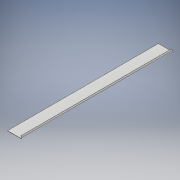
# Autodesk Inventor part: sideplate part 2
Saved by Autodesk Inventor 2018 (Build 220112000, 112)
## iProperties
Created: 2018-06-05
Part Number: sideplate part 2
Material: Generic
Document SubType Name: Sheet Metal
Designer: John Viljoen
Density: 1 g/cm^3
Sheet Metal Rule: Default_mm
Appearance: Default
Author: John Viljoen
Autodesk Inventor part; units mm, degrees
ref_plane "YZ Plane" through (0, 0, 0) normal (1, 0, 0) x (0, 1, 0)
ref_plane "XZ Plane" through (0, 0, 0) normal (0, 1, 0) x (-1, 0, 0)
ref_plane "XY Plane" through (0, 0, 0) normal (0, 0, 1) x (1, 0, 0)
sketch "Sketch1" plane through (0, 0, 0) normal (0, 0, 1) x (1, 0, 0)
  line L0 (0, 0) -> (29.621, 0)
  line L1 (29.621, 0) -> (29.621, 338.525)
  line L2 (29.621, 338.525) -> (0, 338.525)
  line L3 (0, 338.525) -> (0, 0)
  dimension "d0" = 29.621
  dimension "d1" = 338.525
  measures "d0" distance of L2.end L1.end
  measures "d1" distance of L1.end L0.end
extrude "Plate1" add sketch "Sketch1" along normal blind 0.5
sketch "Sketch2" plane through (31.0058, 338.525, 2.5764) normal (0.9232102, 0, 0.3842953) x (0, 1, 0)
  line L0 (-338.525, 0) -> (0, 0)
  line L1 (0, 0) -> (0, 3.0011)
  line L2 (0, 3.0011) -> (-338.525, 3.0011)
  line L3 (-338.525, 3.0011) -> (-338.525, 0)
  constraints: 6 end point, 1 horizontal, 1 perpendicular, 1 vertical
edge flange "Flange1" height 6 angle 112.6 thickness 0.5 bend radius 1.5 thickness toward (0.9232102, 0, 0.3842953) relief straight relief width 0.5 relief depth 0.25 edges at (29.621, 169.2625, 0.5) wall of the first edge with corners at (31.0058, 0, 2.5764) (31.0058, 338.525, 2.5764) (29.8525, 338.525, 5.3471) (29.8525, 0, 5.3471)
bend "Bend1"
corner "Corner1"
equation "\"d2\" = Thickness"
equation "\"d3\" = BendReliefWidth"
equation "\"d4\" = BendReliefDepth"
equation "\"d5\" = MinimumRemnant"
equation "\"d6\" = TransitionRadius"
equation "\"d10\" = CornerReliefSize"
equation "\"d11\" = GapSize"
equation "\"d12\" = JacobiRadiusSize"
equation "\"BendRadius\" = Thickness"
equation "\"BendReliefWidth\" = Thickness"
equation "\"BendReliefDepth\" = 0.5 * Thickness"
equation "\"CornerReliefSize\" = 4 * Thickness"
equation "\"MinimumRemnant\" = 2 * Thickness"
equation "\"TransitionRadius\" = BendRadius"
equation "\"JacobiRadiusSize\" = BendRadius"
equation "\"GapSize\" = Thickness"
equation "\"Thickness\" = 0.5"
body "Solid1"
